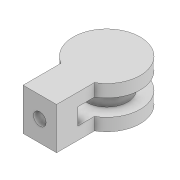
# Autodesk Inventor part: Differential
Saved by Autodesk Inventor 2022 (Build 260153000, 153)
## iProperties
Created: 2022-08-27
Part Number: Differential
Material: Generic
Document SubType Name: Modeling
Designer: dell
Density: 1 g/cm^3
Appearance: Default
Author: dell
Autodesk Inventor part; units mm, degrees
ref_plane "YZ Plane" through (0, 0, 0) normal (1, 0, 0) x (0, 1, 0)
ref_plane "XZ Plane" through (0, 0, 0) normal (0, 1, 0) x (-1, 0, 0)
ref_plane "XY Plane" through (0, 0, 0) normal (0, 0, 1) x (1, 0, 0)
sketch "Sketch1" plane through (0, 0, 0) normal (0, 1, 0) x (-1, 0, 0)
  circle A0 centre (0, 0) radius 4
  dimension "d7" = 8
  constraints: 1 centre point
  measures "d7" diameter of A0
extrude "Extrusion1" add sketch "Sketch1" along normal blind 1.5
sketch "Sketch2" plane through (0, 1.5, 0) normal (0, 1, 0) x (1, 0, 0)
  circle A0 centre (0, 0) radius 2.5
  dimension "d10" = 5
  constraints: 1 centre point, 1 coincident
  measures "d10" diameter of A0
extrude "Extrusion2" add sketch "Sketch2" along normal blind 2
sketch "Sketch3" plane through (0, 3.5, 0) normal (0, 1, 0) x (1, 0, 0)
  circle A0 centre (0, 0) radius 2.5 projected
  circle A1 centre (0, 0) radius 4 projected
extrude "Extrusion3" add sketch "Sketch3" along normal blind 1.5 contours A0 | A1
sketch "Sketch5" plane through (0, 5, 0) normal (0, 1, 0) x (1, 0, 0)
  circle A0 centre (0, 0) radius 2.5 projected
  circle A1 centre (0, 0) radius 4 projected
  circle A2 centre (0, 0) radius 4 projected
  line L0 (2, -3.4641) -> (-2, -3.4641)
  line L1 (-2, -3.4641) -> (-2, -8)
  line L2 (-2, -8) -> (2, -8)
  line L3 (2, -8) -> (2, -3.4641)
  dimension "d15" = 4
  dimension "d16" = 4
  constraints: 8 end point, 2 parallel, 2 point on circle, 1 horizontal, 1 perpendicular
  measures "d15" distance between parallel lines of L1 L3
  measures "d16" distance edge to line of A1 L2
extrude "Extrusion4" add sketch "Sketch5" against normal blind 5 contours A1 L3 L2 L1
sketch "Sketch6" plane through (-2, 5, 8) normal (0, 0, 1) x (1, 0, 0)
  circle A0 centre (2, -2.5) radius 0.75
  line L0 (6, -1.5) -> (-2, -1.5) projected
  point P0 (2, -5)
  point P1 (4, -1.5)
  point P2 (0, -1.5)
  dimension "d21" = 1.5
  dimension "d27" = 1
  constraints: 1 centre point
  measures "d21" diameter of A0
  measures "d27" distance from line of L0 A0.centre
extrude "Extrusion5" cut sketch "Sketch6" against normal blind 4.5
sketch "Sketch8" plane through (2, 5, 8) normal (1, 0, 0) x (0, 0, -1)
  line L0 (4.5359, -1.5) -> (4.5359, -3.5) projected
  line L1 (4.5359, -1.5) -> (4.5359, -3.5)
  line L2 (4.5359, -3.5) -> (2.5359, -3.5)
  line L3 (2.5359, -3.5) -> (2.5359, -1.5)
  line L4 (2.5359, -1.5) -> (4.5359, -1.5)
  point P0 (8, -5)
  dimension "d24" = 2
  constraints: 8 end point, 2 parallel, 1 perpendicular, 1 vertical
  measures "d24" distance of L0.end L2.end
extrude "Extrusion6" cut sketch "Sketch8" against normal blind 4.5
body "Solid1"
